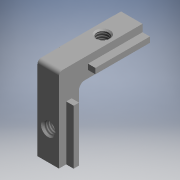
# Autodesk Inventor part: HBLBS5b
Saved by Autodesk Inventor 2017.3 (Build 213256000, 256)
## iProperties
Part Number: HBLBS5b
Material: Generic
Catalog Web Link: www.cadenas.de
Description: HBLBS5b, SHBLBS5b, HBLPBS5b, HABLBS5b, HBLBCA5b, SHBLBCA5b, HBLBCB5b, SHBLBCB5b-Blind Brackets, Sheet Metal Blind Brackets, Post-Assembly Blind Brackets, Corner Blind Brackets(2-Way Type), Corner Blind Brackets(3-Way Type)
Vendor: MISUMI
Document SubType Name: Modeling
Designer: partserver
Manufacturer: MISUMI
Mass: 1.40674 g
Surface Area: 13.237 cm^2
Volume: 1.40674 cm^3
Density: 1 g/cm^3
Appearance: PSOLRGB-192-192-192
Category: PARTsolutions
Company: MISUMI
Title: HBLBS5b
Author: Cadenas PARTsolutions
Comments: Blind Brackets, Sheet Metal Blind Brackets, Post-Assembly Blind Brackets, Corner Blind Brackets(2-Way Type), Corner Blind Brackets(3-Way Type)
PSOL_IDENT_0: {$CADENAS_DATA\23d-libs\misumi\metric\38_al_extrusions_blackets\5\hblbs5.prj},227 {VTYP=3D},{NB=HBLB
PSOL_IDENT_1: S5b},{LINA=HBLBS5b},{NN=HBLBS5b, SHBLBS5b, HBLPBS5b, HABLBS5b, HBLBCA5b, SHBLBCA5b, HBLBCB5b, SHBLBC
PSOL_IDENT_2: B5b},{DATE=18.06.2021 04:10:22},{GEOMDATE=28.05.2021 10:21:27},{VERSION=},{LINEID=60},{WBVAR=},{WBNU
PSOL_IDENT_3: MERIC=}  {NB=HBLBS5b},{LINA=HBLBS5b},{KT=1},{PN=HBLBS5},{VERS=1},{TP=HBLBS5},{MAT=S45C(1045 Steel)(1
PSOL_IDENT_4: .1191_C45E (Ck45))},{ST=Trivalent Chromate},{TYPE=HBLBS5},{MASS=11},{AB=Set Screw M4x5 (Attached)},{
PSOL_IDENT_5: NOB=2},{MATN=-},{MATS=-},{AL=196},{HAB=0.0}
NB: HBLBS5b
NN: HBLBS5b, SHBLBS5b, HBLPBS5b, HABLBS5b, HBLBCA5b, SHBLBCA5b, HBLBCB5b, SHBLBCB5b
NT: Blind Brackets, Sheet Metal Blind Brackets, Post-Assembly Blind Brackets, Corner Blind Brackets(2-Way Type), Corner Blind Brackets(3-Way Type)
NBSYN: $PN.b
LINA: HBLBS5b
CATALOG: Misumi
PN: HBLBS5
MAT: 1045 Carbon Steel
ST: Trivalent Chromate Plating
MASS: 11
AB: Set Screw M4x5 (Attached)
NOB: 2
MATN: -
MATS: -
AL: 196
SUPPLIER: MISUMI
ARTICLENO: HBLBS5b
BOMINFO: HBLBS5b
CREATOR: CADENAS GmbH
Autodesk Inventor part; units mm, degrees
sketch "Sketch_12" plane through (0, 0, 0) normal (0, 0, 1) x (1, 0, 0)
  line L0 (-2.95, 0) -> (2.95, 0)
  line L1 (2.95, 0) -> (2.95, 5.5)
  line L2 (2.95, 5.5) -> (-2.95, 5.5)
  line L3 (-2.95, 5.5) -> (-2.95, 0)
  constraints: 8 end point
extrude "Extrusion1" add sketch "Sketch_12" along normal blind 23
sketch "Sketch_9" plane through (0, 0, 23) normal (0, 0, 1) x (1, 0, 0)
  line L0 (-5, 2) -> (5, 2)
  line L1 (5, 2) -> (5, 3.5)
  line L2 (5, 3.5) -> (-5, 3.5)
  line L3 (-5, 3.5) -> (-5, 2)
  constraints: 8 end point
extrude "Extrusion2" add sketch "Sketch_9" against normal blind 15
sketch "Sketch_8" plane through (0, 0, 0) normal (0, 1, 0) x (-1, 0, 0)
  line L0 (2.95, 5.5) -> (-2.95, 5.5)
  line L1 (-2.95, 5.5) -> (-2.95, 0)
  line L2 (-2.95, 0) -> (2.95, 0)
  line L3 (2.95, 0) -> (2.95, 5.5)
  constraints: 8 end point
extrude "Extrusion3" add sketch "Sketch_8" along normal blind 23
sketch "Sketch_2" plane through (0, 23, 0) normal (0, 1, 0) x (1, 0, 0)
  line L0 (-5, -3.5) -> (5, -3.5)
  line L1 (5, -3.5) -> (5, -2)
  line L2 (5, -2) -> (-5, -2)
  line L3 (-5, -2) -> (-5, -3.5)
  constraints: 8 end point
extrude "Extrusion4" add sketch "Sketch_2" against normal blind 15
sketch "Sketch_4" plane through (0, 0, 0) normal (1, 0, 0) x (0, 1, 0)
  line L0 (5.5, 15) -> (0, 15)
  line L1 (0, 15) -> (0, 17)
  line L2 (0, 17) -> (0.379, 16.621)
  line L3 (0.379, 16.621) -> (5.121, 16.621)
  line L4 (5.121, 16.621) -> (5.5, 17)
  line L5 (5.5, 17) -> (5.5, 15)
  line L6 (5.5, 15) -> (0, 15)
  constraints: 14 end point
revolve "Revolution1" cut sketch "Sketch_4" angle 360 about axis through (0, 5.5, 15) along (0, -1, 0)
thread "Thread1" size "M4x0.7" class "6H" standard "ISO Metric profile" full length
sketch "Sketch_5" plane through (0, 0, 0) normal (1, 0, 0) x (0, 1, 0)
  line L0 (15, 0) -> (15, 5.5)
  line L1 (15, 5.5) -> (17, 5.5)
  line L2 (17, 5.5) -> (16.621, 5.121)
  line L3 (16.621, 5.121) -> (16.621, 0.379)
  line L4 (16.621, 0.379) -> (17, 0)
  line L5 (17, 0) -> (15, 0)
  line L6 (15, 0) -> (15, 5.5)
  constraints: 14 end point
revolve "Revolution2" cut sketch "Sketch_5" angle 360 about axis through (0, 15, 0) along (0, 0, 1)
thread "Thread2" size "M4x0.7" class "6H" standard "ISO Metric profile" full length
sketch "_____1" plane through (0, 0, 0) normal (1, 0, 0) x (0, 0, -1)
  line L0 (-7.1, 5.5) -> (-5.5, 5.5)
  line L1 (-5.5, 5.5) -> (-5.5, 7.1)
  arc A0 (-7.1, 5.5) -> (-5.5, 7.1) centre (-7.1, 7.1) ccw
  constraints: 4 end point, 2 point on circle, 1 centre point
extrude "Extrusion5" add sketch "_____1" along normal mid plane 5.9
sketch "_____2" plane through (0, 0, 0) normal (1, 0, 0) x (0, 0, -1)
  line L0 (-1, 0) -> (0, 0)
  line L1 (0, 0) -> (0, 1)
  arc A0 (-1, 0) -> (0, 1) centre (-1, 1) ccw
  constraints: 4 end point, 2 point on circle, 1 centre point
extrude "Extrusion6" cut sketch "_____2" along normal mid plane 5.9
ref_plane "bracket_to_screw1_XY" through (0, 15, 5) normal (0, 0, -1) x (1, 0, 0)
ref_plane "bracket_to_screw1_YZ" through (0, 15, 5) normal (1, 0, 0) x (0, -1, 0)
ref_plane "bracket_to_screw1_ZX" through (0, 15, 5) normal (0, -1, 0) x (0, 0, -1)
ref_plane "bracket_to_screw2_XY" through (0, 5, 15) normal (0, -1, 0) x (1, 0, 0)
ref_plane "bracket_to_screw2_YZ" through (0, 5, 15) normal (1, 0, 0) x (0, 0, 1)
ref_plane "bracket_to_screw2_ZX" through (0, 5, 15) normal (0, 0, 1) x (0, -1, 0)
body "Solid1"
